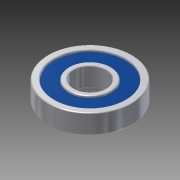
# Autodesk Inventor part: rodamiento
Saved by Autodesk Inventor 2016 (Build 200138000, 138)
## iProperties
Created: 2016-09-08
Part Number: rodamiento
Material: Aluminio 6061
Document SubType Name: Modeling
Designer: Iván
Density: 2.7 g/cm^3
Appearance: Aluminio - Plano
Author: Iván
Autodesk Inventor part; units mm, degrees
ref_plane "YZ Plane" through (0, 0, 0) normal (1, 0, 0) x (0, 1, 0)
ref_plane "XZ Plane" through (0, 0, 0) normal (0, 1, 0) x (-1, 0, 0)
sketch "Boceto1" plane through (0, 0, 0) normal (0, 0, 1) x (1, 0, 0)
  circle A0 centre (0, 0) radius 6.5
  circle A1 centre (0, 0) radius 2.5
  circle A2 centre (0, 0) radius 5.5
  circle A3 centre (0, 0) radius 3.25
  dimension "d0" = 13
  dimension "d1" = 5
  dimension "d2" = 11
  dimension "d3" = 6.5
  constraints: 4 centre point, 4 coincident
  measures "d0" diameter of A0
  measures "d1" diameter of A1
  measures "d2" diameter of A2
  measures "d3" diameter of A3
extrude "Extrusión1" add sketch "Boceto1" along normal blind 3
ref_plane "Plano de trabajo1" through (0, 0, 0.3) normal (0, 0, -1) x (-1, 0, 0)
sketch "Boceto2" plane through (0, 0, 0.3) normal (0, 0, -1) x (-1, 0, 0)
  circle A0 centre (0, 0) radius 3.25
  circle A1 centre (0, 0) radius 5.5
  constraints: 2 centre point, 2 coincident
extrude "Extrusión2" add sketch "Boceto2" against normal blind 2.4
fillet "Empalme1" radius 0.15 8 edges at (-6.5, 0, 3) (-6.5, 0, 0) (-5.5, 0, 3) (-3.25, 0, 3) (-2.5, 0, 3) (-2.5, 0, 0) (-3.25, 0, 0) (-5.5, 0, 0)
